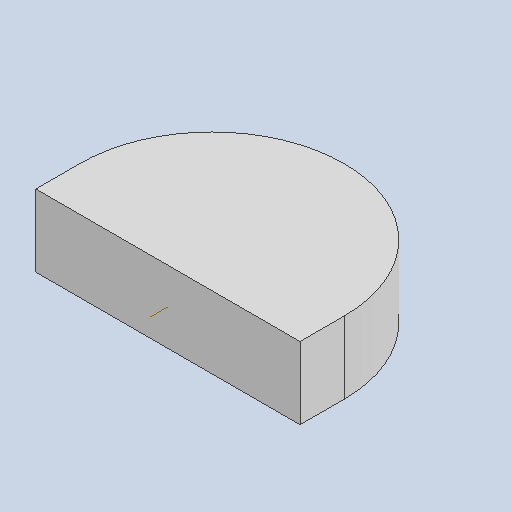
# Autodesk Inventor part: Сыр
Saved by Autodesk Inventor 2023.2 (Build 272271030, 271C)
## iProperties
Created: 2024-01-31
Part Number: Сыр
Material: Типовые
Document SubType Name: Modeling
Designer: I9232
Density: 1 g/cm^3
Appearance: По умолчанию
Author: I9232
Autodesk Inventor part; units mm, degrees
ref_plane "YZ Plane" through (0, 0, 0) normal (1, 0, 0) x (0, 1, 0)
ref_plane "XZ Plane" through (0, 0, 0) normal (0, 1, 0) x (-1, 0, 0)
ref_plane "XY Plane" through (0, 0, 0) normal (0, 0, 1) x (1, 0, 0)
sketch "Эскиз1" plane through (0, 0, 0) normal (0, 1, 0) x (-1, 0, 0)
  line L0 (165, 0.2529) -> (-165, 0.2529)
  line L1 (-165, 0.2529) -> (-165, -54.7471)
  line L2 (165, 0.2529) -> (165, -54.7471)
  arc A0 (-165, -54.7471) -> (165, -54.7471) centre (0, -54.7471) ccw
  point P0 (0, 0)
  dimension "d1" = 330
  dimension "d5" = 55
  dimension "d8" = 55
  constraints: 6 end point, 2 point on circle, 2 tangent, 2 vertical, 1 centre point
  measures "d1" distance of L0.start L0.end
  measures "d5" distance of L0.end L1.end
  measures "d8" distance of L0.start L2.end
extrude "Выдавливание1" add sketch "Эскиз1" along normal mid plane 90
